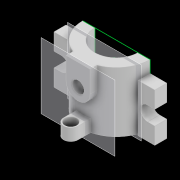
# Autodesk Inventor part: 6-刘宇昂-20202261064
Saved by Autodesk Inventor 2020 (Build 240168000, 168)
## iProperties
Created: 2020-10-16
Part Number: 6-刘宇昂-20202261064
Material: 常规
Document SubType Name: Modeling
Designer: NH55
Density: 1 g/cm^3
Appearance: 默认
Author: NH55
Autodesk Inventor part; units mm, degrees
ref_plane "YZ Plane" through (0, 0, 0) normal (1, 0, 0) x (0, 1, 0)
ref_plane "XZ Plane" through (0, 0, 0) normal (0, 1, 0) x (-1, 0, 0)
sketch "草图1" plane through (0, 0, 0) normal (0, 1, 0) x (-1, 0, 0)
  arc A0 (9, 0) -> (-9, 0) centre (0, 0) ccw
  arc A1 (14, 0) -> (-14, 0) centre (0, 0) ccw
  line L0 (-14, 0) -> (-9, 0)
  line L1 (9, 0) -> (14, 0)
  point P0 (0, 9)
  point P1 (-11.5, 0)
  dimension "d0" = 9
  dimension "d1" = 14
  constraints: 5 point on circle, 4 end point, 2 centre point, 2 coincident, 2 horizontal, 1 collinear, 1 horizontal alignment, 1 midpoint, 1 vertical alignment
  measures "d0" radius of A0
  measures "d1" radius of A1
extrude "拉伸1" add sketch "草图1" along normal blind 25
sketch "草图2" plane through (0, 0, 0) normal (0, 1, 0) x (-1, 0, 0)
  arc A0 (14, 0) -> (-14, 0) centre (0, 0) ccw projected
  line L0 (-14, 0) -> (-9, 0) projected
  arc A1 (9, 0) -> (-9, 0) centre (0, 0) ccw projected
  line L1 (9, 0) -> (14, 0) projected
  arc A2 (14, 0) -> (-14, 0) centre (0, 0) ccw projected
  line L2 (-3, 13.6748) -> (-3, 19)
  arc A3 (3, 19) -> (-3, 19) centre (0, 19) ccw
  line L3 (3, 19) -> (3, 13.6748)
  circle A4 centre (0, 19) radius 2.5
  point P0 (0, 22)
  dimension "d4" = 3
  dimension "d5" = 5
  dimension "d7" = 19
  constraints: 5 point on circle, 4 end point, 2 centre point, 2 tangent, 2 vertical alignment, 1 coincident, 1 parallel, 1 vertical
  measures "d4" radius of A3
  measures "d5" diameter of A4
  measures "d7" distance of point (0, 0) A3.centre
extrude "拉伸2" add sketch "草图2" along normal blind 5 contours A0 L2 A3 L3
ref_plane "工作平面1" through (0, 0, 16) normal (0, 0, 1) x (1, 0, 0)
sketch "草图3" plane through (0, 0, 16) normal (0, 0, 1) x (1, 0, 0)
  line L0 (3, 5) -> (3, 0) projected
  line L1 (3, 0) -> (14, 0) projected
  line L2 (14, 0) -> (14, 25) projected
  line L3 (-14, 25) -> (14, 25) projected
  line L4 (-14, 0) -> (-14, 25) projected
  line L5 (-14, 0) -> (-3, 0) projected
  line L6 (-3, 0) -> (-3, 5) projected
  line L7 (-3, 5) -> (3, 5) projected
  line L8 (-9, 25) -> (9, 25) projected
  line L9 (5, 25) -> (5, 16)
  arc A0 (-5, 16) -> (5, 16) centre (0, 16) ccw
  line L10 (-5, 16) -> (-5, 25)
  circle A1 centre (0, 16) radius 2.5
  line L11 (5, 25) -> (-5, 25)
  point P0 (0, 0)
  point P1 (0, 11)
  point P2 (0, 25)
  dimension "d11" = 5
  dimension "d12" = 9
  dimension "d13" = 5
  constraints: 6 end point, 3 point on circle, 2 centre point, 2 perpendicular, 2 point on line, 2 tangent, 1 coincident, 1 collinear, 1 midpoint, 1 vertical alignment
  measures "d11" radius of A0
  measures "d12" distance of L10.start L10.end
  measures "d13" diameter of A1
extrude "拉伸3" add sketch "草图3" against normal up to surface contours L9 A0 L10 L3
sketch "草图4" plane through (0, 0, 16) normal (0, 0, 1) x (1, 0, 0)
  spline S0 degree 8 poles (2.5, 16) (2.5, 16.2611) (2.4688, 16.5217) (2.4067, 16.7799) (2.313, 17.0334) (2.1864, 17.2794) (2.0254, 17.514) (1.8282, 17.7322) (1.3945, 18.0909) (1.1603, 18.2451) (0.8944, 18.375) (0.6032, 18.4702) (0.2959, 18.5239) (-0.0176, 18.5328) (-0.3266, 18.4972) (-0.9269, 18.3431) (-1.2061, 18.2245) (-1.4564, 18.0745) (-1.6766, 17.8999) (-1.8665, 17.707) (-2.0267, 17.5006) (-2.1582, 17.2852) (-2.3815, 16.8105) (-2.4663, 16.5459) (-2.5169, 16.2746) (-2.5338, 16) (-2.5169, 15.7254) (-2.4663, 15.4541) (-2.3815, 15.1895) (-2.1646, 14.7284) (-2.0431, 14.5264) (-1.8965, 14.3324) (-1.7242, 14.1496) (-1.5254, 13.9819) (-1.3, 13.8342) (-1.0485, 13.712) (-0.5121, 13.5377) (-0.2337, 13.4833) (0.0548, 13.4653) (0.3443, 13.486) (0.6254, 13.5447) (0.8894, 13.6371) (1.1291, 13.7556) (1.641, 14.0805) (1.8946, 14.3104) (2.1011, 14.5662) (2.2627, 14.8391) (2.3818, 15.1227) (2.4605, 15.4126) (2.5, 15.7059) (2.5, 16) knots 0 0 0 0 0 0 0 0 0 0.155112 0.155112 0.155112 0.155112 0.155112 0.155112 0.155112 0.286667 0.286667 0.286667 0.286667 0.286667 0.286667 0.286667 0.422722 0.422722 0.422722 0.422722 0.422722 0.422722 0.422722 0.579191 0.579191 0.579191 0.579191 0.579191 0.579191 0.579191 0.706861 0.706861 0.706861 0.706861 0.706861 0.706861 0.706861 0.827385 0.827385 0.827385 0.827385 0.827385 0.827385 0.827385 1 1 1 1 1 1 1 1 1 projected
  point P0 (0, 0)
  constraints: 1 other
extrude "拉伸4" cut sketch "草图4" against normal up to surface
sketch "草图9" plane through (0, 0, 0) normal (0, 0, 1) x (1, 0, 0)
  line L0 (9, 0) -> (-9, 0) projected
  line L1 (-9, 0) -> (-9, 25) projected
  line L2 (9, 25) -> (-9, 25) projected
  line L3 (9, 0) -> (9, 25) projected
  line L4 (14, 0) -> (9, 0) projected
  line L5 (9, 0) -> (9, 25) projected
  line L6 (14, 25) -> (9, 25) projected
  line L7 (14, 0) -> (14, 25) projected
  line L8 (-9, 0) -> (-14, 0) projected
  line L9 (-14, 0) -> (-14, 25) projected
  line L10 (-9, 25) -> (-14, 25) projected
  line L11 (-9, 0) -> (-9, 25) projected
  point P0 (0, 0)
  constraints: 1 other
ref_plane "工作平面4" through (0, 0, 5) normal (0, 0, 1) x (1, 0, 0)
sketch "草图10" plane through (0, 0, 5) normal (0, 0, 1) x (1, 0, 0)
  line L0 (14, 0) -> (9, 0) projected
  line L1 (9, 0) -> (9, 25) projected
  line L2 (14, 25) -> (9, 25) projected
  line L3 (14, 0) -> (14, 25) projected
  line L4 (9, 0) -> (-9, 0) projected
  line L5 (-9, 0) -> (-9, 25) projected
  line L6 (9, 25) -> (-9, 25) projected
  line L7 (9, 0) -> (9, 25) projected
  line L8 (-9, 0) -> (-14, 0) projected
  line L9 (-14, 0) -> (-14, 25) projected
  line L10 (-9, 25) -> (-14, 25) projected
  line L11 (-9, 0) -> (-9, 25) projected
  line L12 (14, 25) -> (9, 25) projected
  line L13 (14, 25) -> (14, 5)
  line L14 (14, 0) -> (14, 25) projected
  line L15 (-9, 25) -> (-14, 25) projected
  line L16 (-14, 0) -> (-14, 25) projected
  line L17 (14, 0) -> (21, 0)
  line L18 (21, 0) -> (21, 20)
  line L19 (21, 20) -> (14, 20)
  line L20 (-3, 0) -> (-14, 0) projected
  line L21 (-14, 0) -> (-21, 0)
  line L22 (-21, 0) -> (-21, 20)
  line L23 (-21, 20) -> (-14, 20)
  line L24 (21, 13) -> (18, 13)
  arc A0 (18, 13) -> (18, 7) centre (18, 10) ccw
  line L25 (18, 7) -> (21, 7)
  line L26 (-21, 13) -> (-18, 13)
  arc A1 (-18, 7) -> (-18, 13) centre (-18, 10) ccw
  line L27 (-18, 7) -> (-21, 7)
  point P0 (0, 0)
  dimension "d37" = 42
  dimension "d38" = 20
  dimension "d39" = 3
  dimension "d40" = 36
  dimension "d41" = 10
  constraints: 22 end point, 8 point on line, 6 perpendicular, 4 point on circle, 4 tangent, 3 equal length, 3 horizontal, 2 centre point, 1 collinear, 1 equal radius, 1 horizontal alignment, 1 other
  measures "d37" distance of L17.end L21.end
  measures "d38" distance of L17.end L18.end
  measures "d39" radius of A0
  measures "d40" distance of A1.centre A0.centre
  measures "d41" vertical distance of L17.end A0.centre
extrude "拉伸7" add sketch "草图10" against normal up to surface (5 mm away) contours L3 L19 L18 L24 A0 L25 L17 | L21 L22 L27 A1 L26 L23 L9
sketch "草图11" plane through (0, 0, 0) normal (0, -1, 0) x (1, 0, 0)
  point P0 (0, 0)
